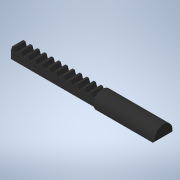
# Autodesk Inventor part: Hammer
Saved by Autodesk Inventor 2021 (Build 250183000, 183)
## iProperties
Created: 2021-03-07
Part Number: Hammer
Material: Generic
Document SubType Name: Modeling
Designer: Lukas
Density: 1 g/cm^3
Appearance: Default
Author: Lukas
Autodesk Inventor part; units mm, degrees
ref_plane "YZ Plane" through (0, 0, 0) normal (1, 0, 0) x (0, 1, 0)
ref_plane "XZ Plane" through (0, 0, 0) normal (0, 1, 0) x (-1, 0, 0)
ref_plane "XY Plane" through (0, 0, 0) normal (0, 0, 1) x (1, 0, 0)
sketch "Sketch5" plane through (0, 0, 0) normal (0, 0, 1) x (1, 0, 0)
  line L0 (-33.5, 0) -> (0, 0)
  line L1 (0, 4.9) -> (0, 0)
  line L2 (-33.5, 4.9) -> (0, 4.9)
  line L3 (-33.5, 4.9) -> (-33.5, 0)
  dimension "d95" = 4.9
  dimension "d106" = 33.5
  constraints: 8 end point, 2 horizontal, 2 vertical
  measures "d95" distance of L1.start L0.end
  measures "d106" distance of L2.start L1.start
revolve "Revolution1" add sketch "Sketch5" angle 360 about axis through (-33.5, 0, 0) along (1, 0, 0)
sketch "Sketch6" plane through (0, 0, 0) normal (1, 0, 0) x (0, 0, -1)
  circle A0 centre (0, 0) radius 4.9 projected
  circle A1 centre (0, 0) radius 4.9 projected
  line L0 (-3.8743, -3) -> (3.8743, -3)
  dimension "d96" = 3
  constraints: 2 end point, 2 point on circle, 1 horizontal
  measures "d96" distance from line of point (0, 0) L0
extrude "Extrusion5" cut sketch "Sketch6" against normal blind 53 contours L0 A0 picked at (-1.032, -3.266)
sketch "Sketch11" plane through (-33.5, 0, 0) normal (0, 0, 1) x (1, 0, 0)
  line L0 (0, -3) -> (0, -3) projected
  line L1 (0, -3) -> (0, 4.9) projected
  line L2 (33.5, -3) -> (0, -3) projected
  line L3 (0, -3) -> (-47, -3)
  line L4 (-47, -3) -> (-47, 3.4)
  line L5 (-47, 3.4) -> (0, 3.4)
  point P0 (33.5, 0)
  dimension "d137" = 47
  dimension "d138" = 6.4
  constraints: 6 end point, 2 perpendicular, 1 horizontal, 1 point on line
  measures "d137" distance of L0.end L3.end
  measures "d138" distance of L3.end L4.end
extrude "Extrusion10" add sketch "Sketch11" along normal mid plane 6
sketch "Sketch12" plane through (-33.5, 0, 3) normal (0, 0, 1) x (1, 0, 0)
  line L0 (-47, -3) -> (0, -3) projected
  line L1 (-47, 3.4) -> (-47, -3) projected
  line L2 (0, 3.4) -> (-47, 3.4) projected
  line L3 (-45.0721, 3.4) -> (-44.3441, 1.4)
  line L4 (-44.3441, 1.4) -> (-43.1441, 1.4)
  line L5 (-43.1441, 1.4) -> (-42.4162, 3.4)
  line L6 (-46.2721, 3.4) -> (-47, 1.4)
  point P0 (33.5, 0)
  dimension "d152" = 1.2
  dimension "d153" = 2
  dimension "d154" = 70
  dimension "d155" = 1.2
  constraints: 8 end point, 4 point on line, 2 equal length, 1 horizontal alignment
  measures "d152" distance of L3.end L4.end
  measures "d153" distance between parallel lines of L2 L4
  measures "d154" angle of L2 L3
  measures "d155" distance of L3.start L6.start
extrude "Extrusion11" cut sketch "Sketch12" against normal through all
pattern_linear "Rectangular Pattern1" count 12 spacing 3.855 along (1, 0, 0) of "Extrusion11"
chamfer "Chamfer5" distance 2 angle 45 1 edges at (0, -3, 0)
body "Solid2"
